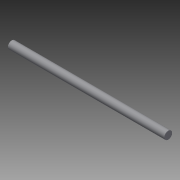
# Autodesk Inventor part: collector Axle
Saved by Autodesk Inventor 2015 (Build 190159000, 159)
## iProperties
Created: 2015-01-27
Part Number: collector Axle
Material: Generic
Document SubType Name: Modeling
Designer: chapale16
Density: 1 g/cm^3
Appearance: Default
Author: chapale16
Autodesk Inventor part; units mm, degrees
ref_plane "YZ Plane" through (0, 0, 0) normal (1, 0, 0) x (0, 1, 0)
ref_plane "XZ Plane" through (0, 0, 0) normal (0, 1, 0) x (-1, 0, 0)
ref_plane "XY Plane" through (0, 0, 0) normal (0, 0, 1) x (1, 0, 0)
sketch "Sketch1" plane through (0, 0, 0) normal (1, 0, 0) x (0, 1, 0)
  circle A0 centre (0, 0) radius 7.62
  dimension "d0" = 15.24
  constraints: 1 centre point, 1 coincident
  measures "d0" diameter of A0
extrude "Extrusion1" add sketch "Sketch1" along normal blind 304.8
body "Solid1"
